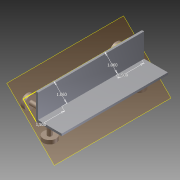
# Autodesk Inventor part: x-bearing assy
Saved by Autodesk Inventor 2012 (Build 160160000, 160)
## iProperties
Created: 2013-05-11
Part Number: x-bearing assy
Material: Default
Document SubType Name: Modeling
Designer: Fabian
Density: 1 g/cm^3
Author: Fabian
Autodesk Inventor part; units mm, degrees
ref_plane "YZ Plane" through (0, 0, 0) normal (1, 0, 0) x (0, 1, 0)
ref_plane "XZ Plane" through (0, 0, 0) normal (0, 1, 0) x (-1, 0, 0)
ref_plane "XY Plane" through (0, 0, 0) normal (0, 0, 1) x (1, 0, 0)
sketch "Sketch1" plane through (0, 0, 0) normal (0, 0, 1) x (1, 0, 0)
  line L0 (-17.5524, 1.6365) -> (20.5476, 1.6365)
  line L1 (20.5476, 1.6365) -> (20.5476, -1.5385)
  line L2 (20.5476, -1.5385) -> (-17.5524, -1.5385)
  line L3 (-17.5524, -1.5385) -> (-17.5524, 1.6365)
  line L4 (-17.5524, -1.5385) -> (-14.3774, -1.5385)
  line L5 (-14.3774, -1.5385) -> (-14.3774, 36.5615)
  line L6 (-14.3774, 36.5615) -> (-17.5524, 36.5615)
  line L7 (-17.5524, 36.5615) -> (-17.5524, -1.5385)
  point P0 (0, 0)
  dimension "d0" = 38.1
  dimension "d1" = 38.1
  dimension "d2" = 3.175
  dimension "d3" = 3.175
  constraints: 16 end point, 4 parallel, 2 horizontal, 2 perpendicular
  measures "d0" distance of L6.end L2.end
  measures "d1" distance of L1.end L2.end
  measures "d2" distance between parallel lines of L7 L5
  measures "d3" distance between parallel lines of L0 L2
extrude "Extrusion1" add sketch "Sketch1" along normal blind 156.21
sketch "Sketch2" plane through (-17.5524, -1.5385, 0) normal (-1, 0, 0) x (0, 0, 1)
  line L0 (156.21, 0) -> (156.21, 38.1) projected
  line L1 (0, 38.1) -> (0, 0) projected
  line L2 (0, 0) -> (156.21, 0) projected
  circle A0 centre (12.7, 7.62) radius 3.175
  circle A1 centre (143.51, 7.62) radius 3.175
  point P0 (0, 1.5385)
  dimension "d6" = 6.35
  dimension "d7" = 6.35
  dimension "d8" = 12.7
  dimension "d9" = 12.7
  dimension "d10" = 7.62
  dimension "d11" = 7.62
  constraints: 2 centre point
  measures "d6" diameter of A0
  measures "d7" diameter of A1
  measures "d8" distance from line of L1 A0.centre
  measures "d9" distance from line of L0 A1.centre
  measures "d10" distance from line of L2 A0.centre
  measures "d11" distance from line of L2 A1.centre
extrude "Extrusion2" add sketch "Sketch2" along normal blind 25.4
sketch "Sketch3" plane through (-17.5524, -1.5385, 0) normal (0, -1, 0) x (1, 0, 0)
  line L0 (38.1, 156.21) -> (0, 156.21) projected
  line L1 (0, 0) -> (0, 156.21) projected
  line L2 (0, 0) -> (38.1, 0) projected
  circle A0 centre (7.62, 143.51) radius 3.175
  circle A1 centre (7.62, 12.7) radius 3.175
  point P0 (17.5524, 0)
  dimension "d14" = 12.7
  dimension "d15" = 12.7
  dimension "d16" = 7.62
  dimension "d17" = 7.62
  dimension "d18" = 6.35
  dimension "d19" = 6.35
  constraints: 2 centre point
  measures "d14" distance from line of L0 A0.centre
  measures "d15" distance from line of L2 A1.centre
  measures "d16" distance from line of L1 A1.centre
  measures "d17" distance from line of L1 A0.centre
  measures "d18" diameter of A0
  measures "d19" diameter of A1
extrude "Extrusion3" add sketch "Sketch3" along normal blind 25.4
sketch "Sketch4" plane through (-42.9524, 6.0815, 143.51) normal (-1, 0, 0) x (0, 0, 1)
  circle A0 centre (0, 0) radius 3.175 projected
  circle A1 centre (0, 0) radius 9.525
  point P0 (-143.51, -6.0815)
  dimension "d22" = 19.05
  constraints: 1 centre point, 1 coincident
  measures "d22" diameter of A1
extrude "Extrusion4" add sketch "Sketch4" against normal blind 5.5372
sketch "Sketch5" plane through (-42.9524, 6.0815, 12.7) normal (-1, 0, 0) x (0, 0, 1)
  circle A0 centre (0, 0) radius 3.175 projected
  circle A1 centre (0, 0) radius 9.525
  point P0 (-12.7, -6.0815)
  dimension "d25" = 19.05
  constraints: 1 centre point, 1 coincident
  measures "d25" diameter of A1
extrude "Extrusion5" add sketch "Sketch5" against normal blind 5.5372
sketch "Sketch6" plane through (-9.9324, -26.9385, 143.51) normal (0, -1, 0) x (1, 0, 0)
  circle A0 centre (0, 0) radius 3.175 projected
  circle A1 centre (0, 0) radius 9.525
  point P0 (9.9324, -143.51)
  dimension "d28" = 19.05
  constraints: 1 centre point, 1 coincident
  measures "d28" diameter of A1
extrude "Extrusion6" add sketch "Sketch6" against normal blind 5.5372
sketch "Sketch7" plane through (-9.9324, -26.9385, 12.7) normal (0, -1, 0) x (1, 0, 0)
  circle A0 centre (0, 0) radius 3.175 projected
  circle A1 centre (0, 0) radius 9.525
  point P0 (9.9324, -12.7)
  dimension "d31" = 19.05
  constraints: 1 centre point, 1 coincident
  measures "d31" diameter of A1
extrude "Extrusion7" add sketch "Sketch7" against normal blind 5.5372
ref_plane "Work Plane1" through (-17.5524, -1.5385, 0) normal (0.7071, 0.7071, 0) x (0, 0, 1)
sketch "Sketch8" plane through (-17.5524, -1.5385, 0) normal (0.7071, 0.7071, 0) x (0, 0, 1)
  line L0 (156.21, 0) -> (156.21, -26.9408) projected
  line L1 (0, -26.9408) -> (0, 0) projected
  line L2 (0, -26.9408) -> (156.21, -26.9408) projected
  point P0 (0, 11.3236)
  point P1 (38.1, -0.0168)
  point P2 (118.11, -0.0168)
  dimension "d35" = 38.1
  dimension "d36" = 38.1
  dimension "d37" = 26.924
  dimension "d38" = 26.924
  measures "d35" distance from line of L0 point (118.11, -0.017)
  measures "d36" distance from line of L1 point (38.1, -0.017)
  measures "d37" distance from line of L2 point (118.11, -0.017)
  measures "d38" distance from line of L2 point (38.1, -0.017)
equation "\"d7\" = d6"
body "Solid1"
